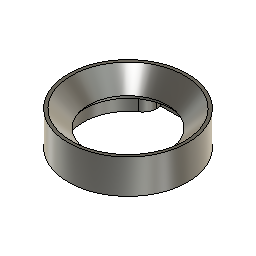
lens bezel v5 (Autodesk Fusion 360 design; units mm, degrees)
Autodesk Fusion 360 part; units mm, degrees
sketch "Sketch1" plane through (0, 0, 0) normal (0, 0, 1) x (1, 0, 0)
  circle A0 centre (0, 0) radius 18.25
  circle A1 centre (0, 0) radius 24.5
  circle A2 centre (0, 0) radius 17.75
  circle A3 centre (0, 0) radius 16.25
  dimension "d1" = 36.5
  dimension "d2" = 49
  dimension "d7" = 35.5
  dimension "d27" = 32.5
  constraint coincident A0.centre A1.centre
  constraint concentric A0 A1
  measures "d1" diameter of A0
  measures "d2" diameter of A1
  measures "d7" diameter of A2
  measures "d27" diameter of A3
extrude "Extrude1" add sketch "Sketch1" along normal blind 15 contours A0 | A1 | A2
extrude "Extrude6" cut sketch "Sketch1" along normal blind 8 contours A2
extrude "Extrude2" cut sketch "Sketch1" along normal blind 6 contours A0
sketch "Sketch5" plane through (0, 0, 0) normal (0, 0, 1) x (1, 0, 0)
  line L0 (-8, 21.5) -> (8, 21.5)
  line L1 (8, 21.5) -> (8, 19.8006)
  line L2 (8, -21.5) -> (-8, -21.5)
  line L3 (-8, 19.8006) -> (-8, 21.5)
  line L4 (-8, 21.5) -> (8, -21.5) construction
  line L5 (8, 21.5) -> (-8, -21.5) construction
  circle A0 centre (0, 0) radius 18.25
  arc A1 (-10.5361, 14.9015) -> (10.5361, 14.9015) centre (0, 0) ccw
  arc A2 (8, 19.8006) -> (10.5361, 14.9015) centre (14, 19.8006) ccw
  arc A3 (-10.5361, 14.9015) -> (-8, 19.8006) centre (-14, 19.8006) ccw
  dimension "d31" = 16
  dimension "d32" = 43
  dimension "d33" = 6
  dimension "d34" = 6
  constraint horizontal L0
  constraint perpendicular L0 L1
  constraint parallel L0 L2
  constraint parallel L1 L3
  constraint coincident L4 A0.centre
  constraint coincident L5 A0.centre
  constraint coincident A0.centre A1.centre
  constraint tangent A1 A2
  constraint tangent L1 A2
  constraint tangent A1 A3
  constraint tangent L3 A3
  measures "d31" distance of L2.start L2.end
  measures "d32" distance of L0.end L2.start
  measures "d33" radius of A2
  measures "d34" radius of A3
extrude "Extrude7" cut sketch "Sketch5" along normal blind 6 contours L0 L1 L3 A0 A2 A3
chamfer "Chamfer3" distance 7 angle 45 1 edges at (-15.1503, 5.8763, 15)
move_face "OffsetFaces1" offset -1 1 faces at (0, -22.371, 0)
